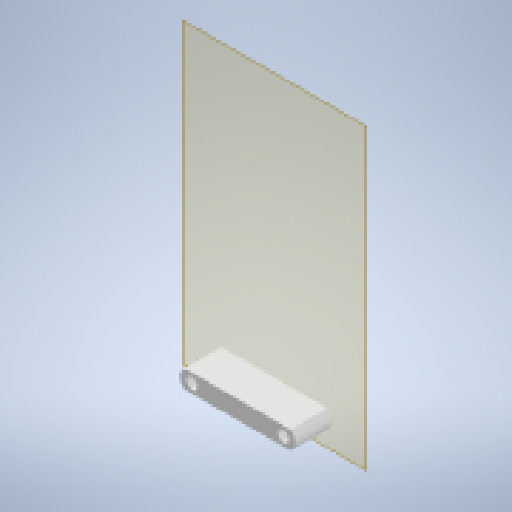
# Autodesk Inventor part: thigh_adt_2
Saved by Autodesk Inventor 2024.3 (Build 283343000, 343)
## iProperties
Created: 2024-09-03
Part Number: thigh_adt_2
Material: PMMA 플라스틱
Document SubType Name: Sheet Metal
Designer: gretc
Density: 1.188 g/cm^3
Sheet Metal Rule: 기본값
Appearance: 주황색-빨간색
Author: gretc
Autodesk Inventor part; units mm, degrees
ref_plane "YZ Plane" through (0, 0, 0) normal (1, 0, 0) x (0, 1, 0)
ref_plane "XZ Plane" through (0, 0, 0) normal (0, 1, 0) x (-1, 0, 0)
ref_plane "XY Plane" through (0, 0, 0) normal (0, 0, 1) x (1, 0, 0)
ref_plane "작업 평면1" through (0, 0, 0) normal (0, 0, 1) x (1, 0, 0)
sketch "스케치1" plane through (0, 0, 0) normal (0, 0, 1) x (1, 0, 0)
  line L0 (13.5, -39.75) -> (11.5, -39.75) projected
  arc A0 (11.5, -39.75) -> (9.25, -42) centre (11.5, -42) ccw projected
  line L1 (9.25, -42) -> (9.25, -44) projected
  arc A1 (8.25, -45) -> (9.25, -44) centre (8.25, -44) ccw projected
  line L2 (8.25, -45) -> (-8.25, -45) projected
  arc A2 (-9.25, -44) -> (-8.25, -45) centre (-8.25, -44) ccw projected
  line L3 (-9.25, -44) -> (-9.25, -42) projected
  arc A3 (-9.25, -42) -> (-11.5, -39.75) centre (-11.5, -42) ccw projected
  line L4 (-11.5, -39.75) -> (-13.5, -39.75) projected
  arc A4 (-14.5, -38.75) -> (-13.5, -39.75) centre (-13.5, -38.75) ccw projected
  line L5 (-14.5, -38.75) -> (-14.5, 8.25) projected
  arc A5 (-13.5, 9.25) -> (-14.5, 8.25) centre (-13.5, 8.25) ccw projected
  line L6 (-13.5, 9.25) -> (-11.5, 9.25) projected
  arc A6 (-11.5, 9.25) -> (-9.25, 11.5) centre (-11.5, 11.5) ccw projected
  line L7 (-9.25, 11.5) -> (-9.25, 14.5) projected
  line L8 (-15, 14.5) -> (-9.25, 14.5) projected
  line L9 (-20.1, 8.5) -> (-15, 14.5) projected
  line L10 (-20.1, -44.6) -> (-20.1, 8.5) projected
  line L11 (-15, -50.6) -> (-20.1, -44.6) projected
  line L12 (15, -50.6) -> (-15, -50.6) projected
  line L13 (20.1, -44.6) -> (15, -50.6) projected
  line L14 (20.1, 8.5) -> (20.1, -44.6) projected
  line L15 (15, 14.5) -> (20.1, 8.5) projected
  line L16 (9.25, 14.5) -> (15, 14.5) projected
  line L17 (9.25, 14.5) -> (9.25, 11.5) projected
  arc A7 (9.25, 11.5) -> (11.5, 9.25) centre (11.5, 11.5) ccw projected
  line L18 (11.5, 9.25) -> (13.5, 9.25) projected
  arc A8 (14.5, 8.25) -> (13.5, 9.25) centre (13.5, 8.25) ccw projected
  line L19 (14.5, 8.25) -> (14.5, -38.75) projected
  arc A9 (13.5, -39.75) -> (14.5, -38.75) centre (13.5, -38.75) ccw projected
  circle A10 centre (17.3, 4) radius 1.35 projected
  circle A11 centre (17.3, -18) radius 1.35 projected
  circle A12 centre (11, -47.8) radius 1.35 projected
  circle A13 centre (-17.3, 4) radius 1.35 projected
  circle A14 centre (-17.3, -18) radius 1.35 projected
  circle A15 centre (-11, -47.8) radius 1.35 projected
  circle A16 centre (17.3, -40) radius 1.35 projected
  circle A17 centre (-17.3, -40) radius 1.35 projected
  arc A18 (12.7321, -50) -> (12.7321, -45.6) centre (11, -47.8) ccw
  line L20 (-10.8997, -45) -> (-7.025, -45) projected
  line L21 (7.025, -45) -> (10.8997, -45) projected
  line L22 (-12.7321, -45.6) -> (12.7321, -45.6)
  line L23 (12.7321, -50) -> (-12.7321, -50)
  arc A19 (-12.7321, -45.6) -> (-12.7321, -50) centre (-11, -47.8) ccw
  arc A20 (-9.2679, -50) -> (-9.25, -49.9857) centre (-11, -47.8) ccw
  arc A21 (-9.25, -45.6143) -> (-9.2679, -45.6) centre (-11, -47.8) ccw
  point P0 (0, 0)
  dimension "d4" = 2.2
  dimension "d5" = 2.2
  dimension "d6" = 103.574
  constraints: 8 point on circle, 4 centre point, 4 end point, 4 point on line, 2 coincident, 2 horizontal, 1 tangent
  measures "d4" distance from line of L22 A19.centre
  measures "d5" distance from line of L23 A15.centre
extrude "돌출1" add sketch "스케치1" along normal blind 8.9 contours L23 A19 L22 A18
equation "\"TransitionRadius\" = BendRadius"
equation "\"BendRadius\" = 2"
